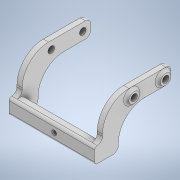
# Autodesk Inventor part: Tendon_Center
Saved by Autodesk Inventor 2021 (Build 250183000, 183)
## iProperties
Created: 2022-10-03
Part Number: Tendon_Center
Material: Generic
Document SubType Name: Modeling
Designer: ereg140
Density: 1 g/cm^3
Appearance: Default
Author: ereg140
Autodesk Inventor part; units mm, degrees
ref_plane "XZ Plane" through (0, 0, 0) normal (0, 1, 0) x (-1, 0, 0)
ref_plane "XY Plane" through (0, 0, 0) normal (0, 0, 1) x (1, 0, 0)
sketch "Sketch1" plane through (0, 0, 0) normal (0, 0, 1) x (1, 0, 0)
  circle A0 centre (-11, 0) radius 1.25 construction
  circle A1 centre (11, 0) radius 1.25 construction
  circle A2 centre (0, -8) radius 12.25 construction
  circle A3 centre (-11, 24) radius 1.5 construction
  circle A4 centre (11, 24) radius 1.5 construction
  line L0 (-14.25, 27.25) -> (14.25, 27.25) construction
  line L1 (14.25, 27.25) -> (14.25, -19.25) construction
  line L2 (14.25, -19.25) -> (-14.25, -19.25) construction
  line L3 (-14.25, -19.25) -> (-14.25, 27.25) construction
  line L4 (-16.25, 10.25) -> (16.25, 10.25)
  line L5 (16.25, 10.25) -> (16.25, 4.25)
  line L6 (16.25, 4.25) -> (-16.25, 4.25)
  line L7 (-16.25, 4.25) -> (-16.25, 10.25)
  circle A5 centre (0.9, 7.25) radius 0.9
  line L8 (0, 4.25) -> (0, 10.25) construction
  circle A6 centre (0, -8) radius 9.5 construction
  point P0 (0, 0)
  point P1 (0, 27.25)
  point P2 (16.25, 7.25)
  dimension "d0" = 2.5
  dimension "d1" = 2.5
  dimension "d2" = 22
  dimension "d3" = 11
  dimension "d4" = 8
  dimension "d5" = 24.5
  dimension "d6" = 3
  dimension "d7" = 3
  dimension "d8" = 24
  dimension "d9" = 28.5
  dimension "d10" = 3.25
  dimension "d11" = 46.5
  dimension "d12" = 2
  dimension "d13" = 6
  dimension "d14" = 1.8
  dimension "d15" = 19
  constraints: 18 end point, 7 centre point, 5 vertical alignment, 4 horizontal alignment, 4 midpoint, 4 parallel, 2 horizontal, 2 perpendicular, 2 tangent, 1 coincident, 1 vertical
  measures "d0" diameter of A0
  measures "d1" diameter of A1
  measures "d2" distance of A1.centre A0.centre
  measures "d3" distance of point (0, 0) A0.centre
  measures "d4" vertical distance of A0.centre A2.centre
  measures "d5" diameter of A2
  measures "d6" diameter of A3
  measures "d7" diameter of A4
  measures "d8" distance of A3.centre A0.centre
  measures "d9" distance between parallel lines of L1 L3
  measures "d10" distance from line of L0 A3.centre
  measures "d11" distance between parallel lines of L2 L0
  measures "d12" distance between parallel lines of L3 L7
  measures "d13" distance between parallel lines of L4 L6
  measures "d14" diameter of A5
  measures "d15" diameter of A6
extrude "Extrusion1" add sketch "Sketch1" along normal blind 3
ref_plane "Work Plane1" through (14.25, 0, 0) normal (1, 0, 0) x (0, 1, 0)
sketch "Sketch2" plane through (14.25, 0, 0) normal (1, 0, 0) x (0, 1, 0)
  line L0 (4.25, 0) -> (10.25, 0) projected
  circle A0 centre (20, -11) radius 1.25
  circle A1 centre (20, -23) radius 1.25
  line L1 (17, -26) -> (23, -26)
  line L2 (23, -26) -> (23, -6)
  line L3 (23, -6) -> (17, -6) construction
  line L4 (17, -6) -> (17, -26)
  line L5 (4.25, 0) -> (23, 0)
  line L6 (23, 0) -> (23, -6)
  line L7 (23, -6) -> (4.25, -6) construction
  line L8 (4.25, -6) -> (4.25, 0)
  line L9 (4.25, -6) -> (17, -6)
  point P0 (0, 0)
  point P1 (27.25, 0)
  point P2 (27.25, 0)
  point P3 (27.25, 0)
  point P4 (20, -26)
  dimension "d19" = 7.25
  dimension "d20" = 11
  dimension "d21" = 12
  dimension "d22" = 2.5
  dimension "d23" = 2.5
  dimension "d24" = 3
  dimension "d25" = 3
  dimension "d26" = 6
  constraints: 18 end point, 4 parallel, 3 perpendicular, 2 centre point, 2 horizontal, 2 vertical alignment, 1 midpoint
  measures "d19" horizontal distance of point (27.25, 0) A0.centre
  measures "d20" vertical distance of point (27.25, 0) A0.centre
  measures "d21" distance of A1.centre A0.centre
  measures "d22" diameter of A0
  measures "d23" diameter of A1
  measures "d24" distance from line of L2 A1.centre
  measures "d25" distance from line of A1.centre L1
  measures "d26" distance between parallel lines of L5 L7
extrude "Extrusion2" add sketch "Sketch2" along normal up to surface (2 mm away)
fillet "Fillet1" radius 10 2 edges at (15.25, 17, -6) (15.25, 23, 0)
fillet "Fillet1" radius 2 4 edges at (15.25, 4.25, -6) (15.25, 17, -26) (15.25, 23, -26) (15.25, 10.25, 0)
mirror "Mirror1" about plane through (0, 0, 0) normal (1, 0, 0) of "Extrusion2", "Fillet1"
fillet "Fillet2" radius 1 2 edges at (0, 10.25, 3) (0, 4.25, 3)
sketch "Sketch3" plane through (-16.25, 19, -26) normal (-1, 0, 0) x (0, 0, 1)
  arc A0 (2, 4) -> (0, 2) centre (2, 2) ccw construction
  line L0 (2, 4) -> (16, 4) construction
  arc A1 (26, -6) -> (16, 4) centre (16, -6) ccw construction
  line L1 (26, -6) -> (26, -6.75) construction
  arc A2 (26, -6.75) -> (28, -8.75) centre (28, -6.75) ccw construction
  arc A3 (29, -9.75) -> (28, -8.75) centre (28, -9.75) ccw construction
  line L2 (29, -9.75) -> (29, -13.75) construction
  arc A4 (28, -14.75) -> (29, -13.75) centre (28, -13.75) ccw construction
  line L3 (28, -14.75) -> (22, -14.75) construction
  arc A5 (20, -12.75) -> (22, -14.75) centre (22, -12.75) ccw construction
  line L4 (20, -12.75) -> (20, -12) construction
  arc A6 (20, -12) -> (10, -2) centre (10, -12) ccw construction
  line L5 (10, -2) -> (2, -2) construction
  arc A7 (0, 0) -> (2, -2) centre (2, 0) ccw construction
  line L6 (0, 0) -> (0, 2) construction
  circle A8 centre (15, 1) radius 1.25 projected
  circle A9 centre (3, 1) radius 1.25 construction
  circle A10 centre (3, 1) radius 1.25 projected
  circle A11 centre (3, 1) radius 2
  circle A12 centre (15, 1) radius 2
  point P0 (26, -19)
  dimension "d32" = 4
  dimension "d33" = 4
  constraints: 2 centre point, 2 coincident
  measures "d32" diameter of A11
  measures "d33" diameter of A12
extrude "Extrusion3" add sketch "Sketch3" along normal blind 1
fillet "Fillet3" radius 1 2 edges at (-16.25, 20, -25) (-16.25, 20, -13)
mirror "Mirror2" about plane through (0, 0, 0) normal (1, 0, 0) of "Extrusion3", "Fillet3"
equation "\"d3\" = 0.5 * d2"
equation "\"d7\" = d6"
equation "\"d23\" = d22"
equation "\"d25\" = d24"
equation "\"d33\" = d32"
body "Solid1"
